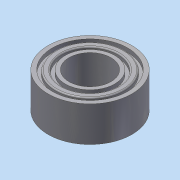
# Autodesk Inventor part: Mini Bearing
Saved by Autodesk Inventor 2013 (Build 170138000, 138)
## iProperties
Created: 2013-06-21
Part Number: Mini Bearing
Material: Steel
Document SubType Name: Modeling
Designer: Jon Hollander
Mass: 1.4501 g
Surface Area: 2.7269 cm^2
Volume: 0.184726 cm^3
Density: 7.85 g/cm^3
Author: Jon Hollander
Autodesk Inventor part; units mm, degrees
ref_plane "YZ Plane" through (0, 0, 0) normal (1, 0, 0) x (0, 1, 0)
ref_plane "XZ Plane" through (0, 0, 0) normal (0, 1, 0) x (-1, 0, 0)
ref_plane "XY Plane" through (0, 0, 0) normal (0, 0, 1) x (1, 0, 0)
sketch "Sketch1" plane through (0, 0, 0) normal (0, 0, 1) x (1, 0, 0)
  circle A0 centre (0, 0) radius 5
  circle A1 centre (0, 0) radius 2.5
  dimension "d0" = 10
  dimension "d1" = 5
  constraints: 2 centre point, 2 coincident
  measures "d0" diameter of A0
  measures "d1" diameter of A1
extrude "Extrusion1" add sketch "Sketch1" along normal mid plane 4.2
sketch "Sketch2" plane through (0, 0, 2.1) normal (0, 0, 1) x (1, 0, 0)
  circle A0 centre (0, 0) radius 2.5 projected
  circle A1 centre (0, 0) radius 5 projected
  circle A2 centre (0, 0) radius 4.5
  circle A3 centre (0, 0) radius 4.1
  circle A4 centre (0, 0) radius 2.95
  circle A5 centre (0, 0) radius 3.35
  dimension "d4" = 0.5
  dimension "d5" = 0.4
  dimension "d6" = 0.75
  dimension "d7" = 0.4
  constraints: 4 centre point, 4 coincident
  measures "d4" radial gap between concentric circles of A1 A2
  measures "d5" radial gap between concentric circles of A2 A3
  measures "d6" radial gap between concentric circles of A3 A5
  measures "d7" radial gap between concentric circles of A5 A4
extrude "Extrusion2" cut sketch "Sketch2" against normal blind 0.5 contours A2 | A5
fillet "Fillet1" radius 0.15 2 edges at (-4.1, 0, 2.1) (-3.35, 0, 2.1)
mirror "Mirror1" about plane through (0, 0, 0) normal (0, 0, 1) of "Extrusion2"
fillet "Fillet2" radius 0.15 2 edges at (-4.1, 0, -2.1) (-3.35, 0, -2.1)
body "Solid1"
